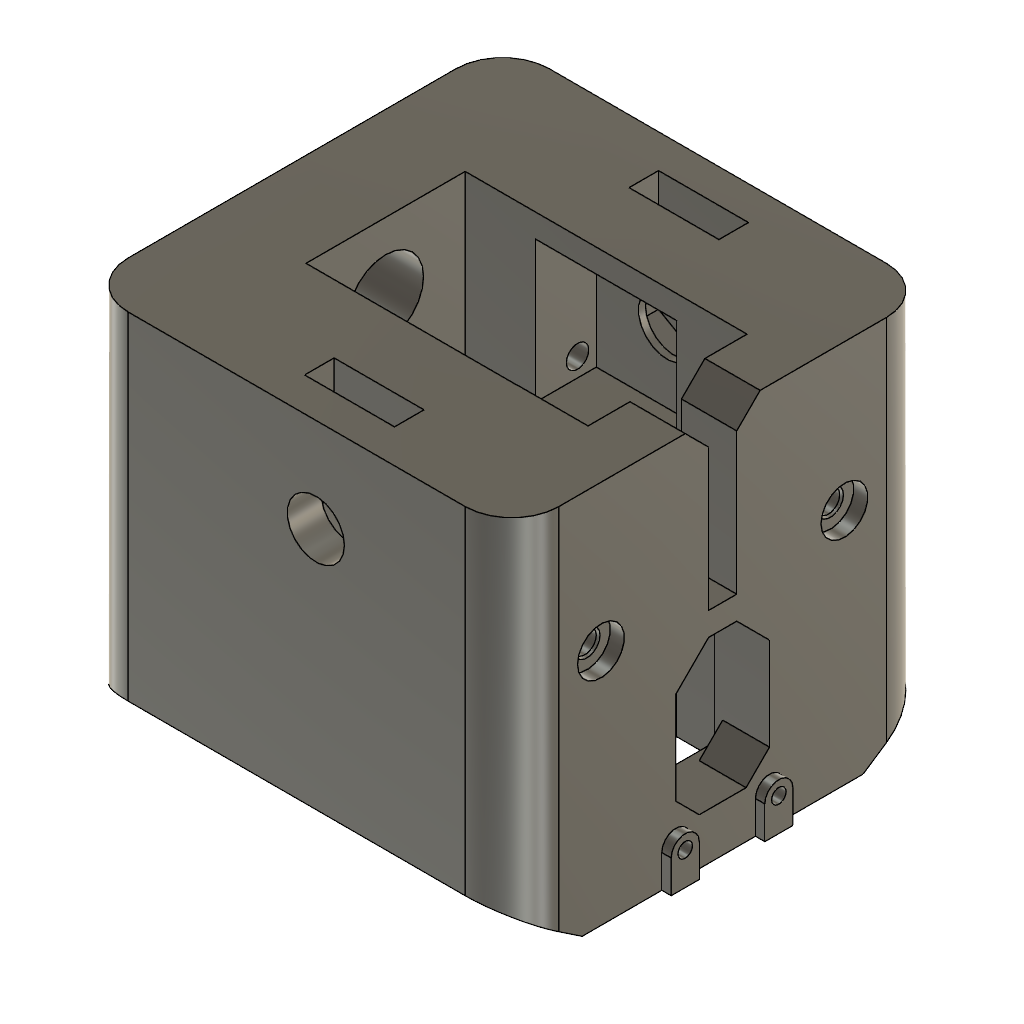
Agarre móvil v40 (Autodesk Fusion 360 design; units mm, degrees)
Autodesk Fusion 360 part; units mm, degrees
sketch "Sketch1" plane through (0, 0, 0) normal (0, 0, 1) x (1, 0, 0)
  line L0 (0, 0) -> (92, 0)
  line L1 (92, 0) -> (92, 60)
  line L2 (92, 60) -> (0, 60)
  line L3 (0, 60) -> (0, 0)
  dimension "d17" = 92
  dimension "d130" = 60
  constraint horizontal L0
  constraint vertical L1
  constraint horizontal L2
  constraint vertical L3
  constraint coincident L0.start L3.end
  measures "d17" distance of L1 L3
  measures "d130" distance of L0 L2
extrude "Extrude1" add sketch "Sketch1" along normal blind 10
sketch "Sketch3" plane through (0, 0, 10) normal (0, 0, 1) x (-1, 0, 0)
  line L0 (0, 0) -> (-92, 0)
  line L1 (-92, 0) -> (-92, -60)
  line L2 (-92, -60) -> (0, -60)
  line L3 (-92, -75) -> (0, -75)
  line L4 (0, -75) -> (0, 15)
  line L5 (0, 15) -> (-92, 15)
  line L6 (-92, 15) -> (-92, -75)
  line L7 (-20, -40) -> (-92, -40)
  line L8 (-92, -40) -> (-92, -20)
  line L9 (-92, -20) -> (-20, -20)
  line L10 (-20, -20) -> (-20, -40)
  line L11 (0, -60) -> (0, 0)
  dimension "d58" = 15
  dimension "d59" = 15
  dimension "d134" = 20
  constraint horizontal L3
  constraint vertical L4
  constraint horizontal L5
  constraint vertical L6
  constraint horizontal L7
  constraint vertical L8
  constraint horizontal L9
  constraint vertical L10
  constraint coincident L6 L8.end
  constraint coincident L1 L8.end
  measures "d58" distance of L2 L3
  measures "d59" distance of L0 L5
  measures "d134" distance of L7 L9
extrude "Extrude3" add sketch "Sketch3" along normal blind 72 contours L0 L1 L2 L4 L6 L7 L9 L10 L11 | L0 L4 L5 L6 | L2 L3 L4 L6
sketch "Sketch4" plane through (20, 0, 0) normal (1, 0, 0) x (0, 1, 0)
  line L0 (20, 82) -> (20, 10)
  line L1 (20, 10) -> (40, 10)
  line L2 (40, 10) -> (40, 82)
  line L3 (40, 82) -> (20, 82)
  circle A0 centre (30, 67) radius 8.1
  dimension "d7" = 16.2
  dimension "d8" = 15
  measures "d7" diameter of A0
  measures "d8" distance of L3 A0.centre
extrude "Extrude4" cut sketch "Sketch4" against normal blind 20 contours A0
sketch "Sketch5" plane through (0, 20, 0) normal (0, 1, 0) x (-1, 0, 0)
  line L0 (-92, 10) -> (-20, 10)
  line L1 (-20, 10) -> (-20, 82)
  line L2 (-20, 82) -> (-92, 82)
  line L3 (-92, 82) -> (-92, 10)
  line L4 (-65.2, 77) -> (-35, 77)
  line L5 (-35, 77) -> (-35, 46.8)
  line L6 (-35, 46.8) -> (-65.2, 46.8)
  line L7 (-65.2, 46.8) -> (-65.2, 77)
  dimension "d11" = 30.2
  dimension "d12" = 30.2
  dimension "d18" = 26.8
  dimension "d67" = 5
  constraint horizontal L4
  constraint vertical L5
  constraint horizontal L6
  constraint vertical L7
  measures "d11" distance of L5 L7
  measures "d12" distance of L4 L6
  measures "d18" distance of L3 L7
  measures "d67" distance of L2 L4
extrude "Extrude5" cut sketch "Sketch5" along normal blind 40 and the other way blind 20 contours L4 L5 L6 L7
sketch "Sketch6" plane through (20, 0, 0) normal (1, 0, 0) x (0, 1, 0)
  circle A0 centre (30, 67) radius 8.1
  line L0 (20, 82) -> (20, 10)
  line L1 (20, 10) -> (40, 10)
  line L2 (40, 10) -> (40, 82)
  line L3 (40, 82) -> (20, 82)
  line L4 (13, 82) -> (47, 82)
  line L5 (47, 82) -> (47, 46.8)
  line L6 (47, 46.8) -> (13, 46.8)
  line L7 (13, 46.8) -> (13, 82)
  dimension "d68" = 35.2
  dimension "d93" = 7
  dimension "d94" = 7
  constraint horizontal L4
  constraint vertical L5
  constraint horizontal L6
  constraint vertical L7
  constraint collinear L3 L4
  measures "d68" distance of L4 L6
  measures "d93" distance of L2 L5
  measures "d94" distance of L0 L7
extrude "Extrude6" cut sketch "Sketch6" along normal blind 45.2 contours L0 L4 L6 L7 | L2 L4 L5 L6
sketch "Sketch7" plane through (65.2, 0, 0) normal (-1, 0, 0) x (0, -1, 0)
  line L0 (-47, 77) -> (-60, 77)
  line L1 (-60, 77) -> (-60, 46.8)
  line L2 (-60, 46.8) -> (-40, 46.8)
  line L3 (-40, 46.8) -> (-40, 82)
  line L4 (-47, 82) -> (-47, 77)
  line L5 (-40, 82) -> (-33, 82)
  line L6 (-33, 82) -> (-33, 46.8)
  line L7 (-33, 46.8) -> (-40, 46.8)
  line L8 (-40, 46.8) -> (-40, 82)
  line L9 (-20, 82) -> (-27, 82)
  line L10 (-27, 82) -> (-27, 46.8)
  line L11 (-27, 46.8) -> (-20, 46.8)
  line L12 (-20, 46.8) -> (-20, 82)
  line L13 (-27, 46.8) -> (-16.8934, 46.8) construction
  line L14 (-20, 10) -> (-20, 82)
  line L15 (-40, 10) -> (-40, 82)
  line L16 (-40, 82) -> (-47, 82)
  line L17 (15, 82) -> (-20, 82)
  line L18 (-20, 46.8) -> (-40, 46.8)
  line L19 (-40, 46.8) -> (-40, 41.8)
  line L20 (-40, 41.8) -> (-20, 41.8)
  line L21 (-20, 41.8) -> (-20, 46.8)
  line L22 (-27, 41.8) -> (-20, 34.8)
  line L23 (-33, 41.8) -> (-40, 34.8)
  dimension "d22" = 7
  dimension "d23" = 7
  dimension "d69" = 35.2
  dimension "d70" = 35.2
  dimension "d101" = 45
  dimension "d102" = 7
  dimension "d103" = 5
  dimension "d104" = 7
  dimension "d131" = 45
  constraint horizontal L5
  constraint vertical L6
  constraint horizontal L7
  constraint vertical L8
  constraint coincident L3.end L5.start
  constraint horizontal L9
  constraint vertical L10
  constraint horizontal L11
  constraint vertical L12
  constraint horizontal L13
  constraint collinear L9 L17
  constraint horizontal L18
  constraint vertical L19
  constraint horizontal L20
  constraint vertical L21
  constraint coincident L15 L19.end
  constraint coincident L14 L22.end
  constraint coincident L20 L22.start
  constraint coincident L20 L23.start
  constraint coincident L15 L23.end
  measures "d22" distance of L10 L12
  measures "d23" distance of L6 L8
  measures "d69" distance of L9.end L10.end
  measures "d70" distance of L5.end L6.end
  measures "d101" angle of L20 L22
  measures "d102" distance of L14 L22.start
  measures "d103" distance of L10.end L20
  measures "d104" distance of L19.end L23.start
  measures "d131" angle of L15 L23
extrude "Extrude7" add sketch "Sketch7" against normal blind 26.8 contours L3 L5 L6 L7 L8 L15 L18 | L7 L11 L14 L15 L18 L19 L20 L21 | L15 L20 L23 | L9 L10 L11 L12 L14 L18 | L14 L20 L22
sketch "Sketch17" plane through (0, 0, 46.8) normal (0, 0, 1) x (-1, 0, 0)
  line L0 (-65.2, -33) -> (-65.2, -27)
  line L1 (-65.2, -27) -> (-92, -27)
  line L2 (-92, -27) -> (-92, -33)
  line L3 (-92, -33) -> (-65.2, -33)
  line L4 (-65.2, -33) -> (-75.2, -33)
  line L5 (-75.2, -33) -> (-75.2, -27)
  line L6 (-75.2, -27) -> (-65.2, -27)
  line L7 (-65.2, -27) -> (-65.2, -33)
  dimension "d105" = 10
  constraint horizontal L4
  constraint vertical L5
  constraint horizontal L6
  constraint vertical L7
  constraint coincident L0.start L3.end
  measures "d105" distance of L0.start L4.end
extrude "Extrude18" cut sketch "Sketch17" against normal blind 6 contours L0 L1 L3 L4 L5 L6 L7
chamfer "Chamfer5" distance 4 angle 45 1 edges at (75.2, 30, 46.8)
sketch "Sketch8" plane through (0, 0, 10) normal (0, 0, 1) x (-1, 0, 0)
  line L0 (-20, -20) -> (-92, -20)
  line L1 (-92, -20) -> (-92, -40)
  line L2 (-92, -40) -> (-20, -40)
  line L3 (-20, -40) -> (-20, -20)
  circle A0 centre (-30, -40) radius 1.6
  circle A1 centre (-50, -40) radius 1.6
  circle A2 centre (-30, -20) radius 1.6
  circle A3 centre (-50, -20) radius 1.6
  dimension "d28" = 3.2
  dimension "d29" = 3.2
  dimension "d30" = 3.2
  dimension "d31" = 3.2
  dimension "d32" = 20
  dimension "d33" = 20
  dimension "d34" = 10
  dimension "d35" = 10
  dimension "d132" = 20
  constraint coincident L2 A0.centre
  constraint coincident L2 A1.centre
  constraint coincident L0 A3.centre
  measures "d28" diameter of A0
  measures "d29" diameter of A1
  measures "d30" diameter of A2
  measures "d31" diameter of A3
  measures "d32" distance of A2.centre A3.centre
  measures "d33" distance of A0.centre A1.centre
  measures "d34" distance of L3 A0.centre
  measures "d35" distance of L3 A2.centre
  measures "d132" distance of A0.centre A2.centre
extrude "Extrude8" cut sketch "Sketch8" against normal blind 10 contours L0 A2 | L0 A2 | L2 A0 | L2 A0 | L0 A3 | L0 A3 | L2 A1 | L2 A1
sketch "Sketch9" plane through (0, 0, 10) normal (0, 0, 1) x (-1, 0, 0)
  arc A0 (-48.4, -40) -> (-51.6, -40) centre (-50, -40) ccw
  line L0 (-48.4, -40) -> (-31.6, -40)
  arc A1 (-28.4, -40) -> (-31.6, -40) centre (-30, -40) ccw
  line L1 (-28.4, -40) -> (-20, -40)
  line L2 (-20, -40) -> (-20, -20)
  line L3 (-20, -20) -> (-28.4, -20)
  arc A2 (-31.6, -20) -> (-28.4, -20) centre (-30, -20) ccw
  line L4 (-31.6, -20) -> (-48.4, -20)
  arc A3 (-51.6, -20) -> (-48.4, -20) centre (-50, -20) ccw
  line L5 (-51.6, -20) -> (-92, -20)
  line L6 (-92, -20) -> (-92, -40)
  line L7 (-92, -40) -> (-51.6, -40)
  circle A4 centre (-30, -40) radius 3
  circle A5 centre (-50, -40) radius 3
  circle A6 centre (-50, -20) radius 3
  circle A7 centre (-30, -20) radius 3
  dimension "d38" = 6
  dimension "d39" = 6
  dimension "d40" = 6
  dimension "d41" = 6
  constraint concentric A1 A4
  constraint concentric A0 A5
  constraint concentric A3 A6
  constraint concentric A2 A7
  measures "d38" diameter of A4
  measures "d39" diameter of A5
  measures "d40" diameter of A6
  measures "d41" diameter of A7
chamfer "Chamfer8" distance 15 distance2 10 2 edges at (46, 0, 10) (46, 60, 10) measured on face at (30.6667, -5, 10) measured on face at (61.3333, 65, 10)
chamfer "Chamfer9" distance 5 angle 45 2 edges at (78.6, 33, 82) (78.6, 27, 82)
extrude "Extrude9" cut sketch "Sketch9" along normal blind 41.8 contours A0 L0 L7 A5 | L0 A1 L1 A4 | L4 A3 L5 A6 | L3 A2 L4 A7 picked at (-50.0747, -40.9972) picked at (-29.9253, -40.9972) picked at (-49.9253, -19.0028) picked at (-29.9253, -19.0028)
sketch "Sketch10" plane through (0, 0, 0) normal (0, 1, 0) x (-1, 0, 0)
  line L0 (-65.2, 46.8) -> (-35, 46.8)
  line L1 (-35, 46.8) -> (-35, 77)
  line L2 (-35, 77) -> (-65.2, 77)
  line L3 (-65.2, 77) -> (-65.2, 46.8)
  circle A0 centre (-50.1, 61.9) radius 6.1
  dimension "d46" = 12.2
  dimension "d47" = 15.1
  dimension "d48" = 15.1
  measures "d46" diameter of A0
  measures "d47" distance of L2 A0.centre
  measures "d48" distance of L3 A0.centre
extrude "Extrude10" cut sketch "Sketch10" along normal blind 75 and the other way blind 15 contours A0
ref_plane "WorkPlane1" through (50.1, -1.5, 61.9) normal (0, 1, 0) x (0, 0, 1)
sketch "Sketch11" plane through (45.1, -1.5, 54.9) normal (0, 1, 0) x (1, 0, 0)
  circle A0 centre (5, -7) radius 6.1
  circle A1 centre (5, -7) radius 6.1
  line L0 (14.6, -1.4574) -> (5, 4.0851)
  line L1 (5, 4.0851) -> (-4.6, -1.4574)
  line L2 (-4.6, -1.4574) -> (-4.6, -12.5426)
  line L3 (-4.6, -12.5426) -> (5, -18.0851)
  line L4 (5, -18.0851) -> (14.6, -12.5426)
  line L5 (14.6, -12.5426) -> (14.6, -1.4574)
  line L6 (14.6, -1.4574) -> (-4.6, -1.4574)
  line L7 (-4.6, -1.4574) -> (-4.6, -28.6763)
  line L8 (-4.6, -28.6763) -> (14.6, -28.6763)
  line L9 (14.6, -28.6763) -> (14.6, -1.4574)
  point P0 (5, -7)
  point P1 (5, -7)
  point P2 (5, -7)
  point P3 (5, -7)
  dimension "d128" = 9.6
  constraint coincident P3 P0
  constraint coincident P1 P0
  constraint coincident P2 P1
  constraint horizontal L6
  constraint vertical L7
  constraint horizontal L8
  constraint vertical L9
  measures "d128" distance of P3 L5
extrude "Extrude11" cut sketch "Sketch11" against normal blind 6.3
ref_plane "WorkPlane2" through (50.1, 61.5, 61.9) normal (0, -1, 0) x (0, 0, -1)
sketch "Sketch12" plane through (45.1, 61.5, 54.9) normal (0, -1, 0) x (1, 0, 0)
  circle A0 centre (5, 7) radius 6.1
  line L0 (14.6, 12.5426) -> (5, 18.0851)
  line L1 (5, 18.0851) -> (-4.6, 12.5426)
  line L2 (-4.6, 12.5426) -> (-4.6, 1.4574)
  line L3 (-4.6, 1.4574) -> (5, -4.0851)
  line L4 (5, -4.0851) -> (14.6, 1.4574)
  line L5 (14.6, 1.4574) -> (14.6, 12.5426)
  line L6 (-4.6, 1.4574) -> (14.6, 1.4574)
  line L7 (14.6, 1.4574) -> (14.6, 28.1341)
  line L8 (14.6, 28.1341) -> (-4.6, 28.1341)
  line L9 (-4.6, 28.1341) -> (-4.6, 1.4574)
  point P0 (5, 7)
  point P1 (5, 7)
  dimension "d95" = 9.6
  constraint coincident P0 A0.centre
  constraint coincident P1 P0
  constraint horizontal L6
  constraint vertical L7
  constraint horizontal L8
  constraint vertical L9
  measures "d95" distance of P1 L5
extrude "Extrude12" cut sketch "Sketch12" against normal blind 6.3 contours A0 L0 L1 L2 L5 L6 L7 L9 | A0 L3 L4 L6 | L0 L1 L7 L8 L9
sketch "Sketch13" plane through (92, 0, 0) normal (1, 0, 0) x (0, 1, 0)
  line L0 (75, 82) -> (38, 82)
  line L1 (40, 34.8) -> (40, 10)
  line L2 (40, 10) -> (20, 10)
  line L3 (20, 10) -> (20, 34.8)
  line L4 (0, 0) -> (60, 0)
  circle A0 centre (20, 7) radius 1.55
  circle A1 centre (40, 7) radius 1.55
  circle A2 centre (20, 7) radius 3
  circle A3 centre (40, 7) radius 3
  line L5 (17, 7) -> (17, 0)
  line L6 (23, 7) -> (23, 0)
  line L7 (37, 7) -> (37, 0)
  line L8 (43, 7) -> (43, 0)
  line L9 (33, 77) -> (33, 46.8)
  line L10 (27, 46.8) -> (27, 77)
  line L11 (33, 46.8) -> (27, 46.8)
  line L12 (20, 34.8) -> (27, 41.8)
  line L13 (27, 41.8) -> (33, 41.8)
  line L14 (33, 41.8) -> (40, 34.8)
  line L15 (22, 82) -> (-15, 82)
  line L16 (-15, 82) -> (-15, 10)
  line L17 (75, 10) -> (75, 82)
  line L18 (27, 77) -> (22, 82)
  line L19 (-15, 10) -> (0, 0)
  line L20 (60, 0) -> (75, 10)
  line L21 (38, 82) -> (33, 77)
  dimension "d71" = 3.1
  dimension "d72" = 3.1
  dimension "d73" = 20
  dimension "d74" = 7
  dimension "d75" = 6
  dimension "d76" = 6
  constraint concentric A0 A2
  constraint concentric A1 A3
  constraint coincident A2 L5.start
  constraint coincident L4 L5.end
  constraint tangent A2 L5
  constraint perpendicular L4 L5
  constraint coincident A2 L6.start
  constraint coincident L4 L6.end
  constraint tangent A2 L6
  constraint perpendicular L4 L6
  constraint coincident L4 L7.end
  constraint perpendicular L4 L7
  constraint coincident A3 L8.start
  constraint coincident L4 L8.end
  constraint tangent A3 L8
  constraint perpendicular L4 L8
  constraint coincident A3 L7.start
  measures "d71" diameter of A0
  measures "d72" diameter of A1
  measures "d73" distance of A0.centre A1.centre
  measures "d74" distance of L4 A0.centre
  measures "d75" diameter of A2
  measures "d76" diameter of A3
extrude "Extrude13" add sketch "Sketch13" along normal blind 2 contours L4 A3 L7 L8 | A3 | L4 A2 L5 L6 | A2
extrude "Extrude14" cut 2 faces at (92, 20.1888, 7.481) (92, 39.3809, 6.5283) along direction (-1, 0, 0) blind 7
sketch "Sketch15" plane through (92, 0, 0) normal (1, 0, 0) x (0, 1, 0)
  line L0 (17, 0) -> (17, 7)
  arc A0 (20, 10) -> (17, 7) centre (20, 7) ccw
  line L1 (20, 10) -> (20, 34.8)
  line L2 (75, 82) -> (38, 82)
  line L3 (43, 0) -> (60, 0)
  line L4 (37, 0) -> (37, 7)
  arc A1 (40, 10) -> (37, 7) centre (40, 7) ccw
  line L5 (40, 10) -> (20, 10)
  arc A2 (23, 7) -> (20, 10) centre (20, 7) ccw
  line L6 (23, 7) -> (23, 0)
  line L7 (23, 0) -> (37, 0)
  line L8 (43, 7) -> (43, 0)
  line L9 (43, 0) -> (60, 0)
  line L10 (75, 82) -> (38, 82)
  line L11 (40, 34.8) -> (40, 10)
  arc A3 (43, 7) -> (40, 10) centre (40, 7) ccw
  line L12 (20, 15) -> (25, 10)
  line L13 (20, 15) -> (27.0711, 15) construction
  line L14 (40, 15) -> (35, 10)
  line L15 (27, 46.8) -> (27, 77)
  line L16 (33, 77) -> (33, 46.8)
  line L17 (43, 7) -> (43, 0)
  line L18 (33, 77) -> (33, 46.8)
  line L19 (33, 46.8) -> (27, 46.8)
  line L20 (40, 34.8) -> (40, 10)
  arc A4 (43, 7) -> (40, 10) centre (40, 7) ccw
  line L21 (33, 46.8) -> (27, 46.8)
  line L22 (27, 46.8) -> (27, 77)
  line L23 (17, 0) -> (17, 7)
  arc A5 (20, 10) -> (17, 7) centre (20, 7) ccw
  line L24 (20, 10) -> (20, 34.8)
  line L25 (20, 34.8) -> (27, 41.8)
  line L26 (20, 34.8) -> (27, 41.8)
  line L27 (27, 41.8) -> (33, 41.8)
  line L28 (33, 41.8) -> (40, 34.8)
  line L29 (27, 41.8) -> (33, 41.8)
  line L30 (33, 41.8) -> (40, 34.8)
  line L31 (75, 10) -> (75, 82)
  line L32 (22, 82) -> (-15, 82)
  line L33 (-15, 82) -> (-15, 10)
  line L34 (75, 10) -> (75, 82)
  line L35 (22, 82) -> (-15, 82)
  line L36 (-15, 82) -> (-15, 10)
  line L37 (60, 0) -> (75, 10)
  line L38 (38, 82) -> (33, 77)
  line L39 (27, 77) -> (22, 82)
  line L40 (-15, 10) -> (0, 0)
  line L41 (0, 0) -> (17, 0)
  line L42 (60, 0) -> (75, 10)
  line L43 (38, 82) -> (33, 77)
  line L44 (27, 77) -> (22, 82)
  line L45 (-15, 10) -> (0, 0)
  line L46 (0, 0) -> (17, 0)
  dimension "d86" = 45
  constraint horizontal L13
  constraint coincident L1 L12.start
  constraint coincident L5 L12.end
  constraint coincident L11 L14.start
  constraint coincident L5 L14.end
  constraint perpendicular L12 L14
  measures "d86" angle of L12 L13
extrude "Extrude16" add sketch "Sketch15" against normal blind 10 contours L1 L5 L12 L24 | L5 L11 L14 L20
ref_plane "WorkPlane3" through (86, 20, 7) normal (1, 0, 0) x (0, 1, 0)
sketch "Sketch14" plane through (86, 20, 7) normal (1, 0, 0) x (0, 1, 0)
  line L0 (2.85, 1.6454) -> (0, 3.2909)
  line L1 (0, 3.2909) -> (-2.85, 1.6454)
  line L2 (-2.85, 1.6454) -> (-2.85, -1.6454)
  line L3 (-2.85, -1.6454) -> (0, -3.2909)
  line L4 (0, -3.2909) -> (2.85, -1.6454)
  line L5 (2.85, -1.6454) -> (2.85, 1.6454)
  line L6 (17.1705, -1.6805) -> (20.0406, -3.2906)
  line L7 (20.0406, -3.2906) -> (22.8701, -1.6102)
  line L8 (22.8701, -1.6102) -> (22.8295, 1.6805)
  line L9 (22.8295, 1.6805) -> (19.9594, 3.2906)
  line L10 (19.9594, 3.2906) -> (17.1299, 1.6102)
  line L11 (17.1299, 1.6102) -> (17.1705, -1.6805)
  line L12 (-2.85, -1.6454) -> (-2.85, -7)
  line L13 (2.85, -1.6454) -> (2.85, -7)
  line L14 (17.1705, -1.6805) -> (22.8498, -1.6805)
  line L15 (22.8498, -1.6805) -> (22.8498, -7.3381)
  line L16 (22.8498, -7.3381) -> (17.1705, -7.3381)
  line L17 (17.1705, -7.3381) -> (17.1705, -1.6805)
  line L18 (2.85, -7) -> (-2.85, -7)
  point P0 (20, 0)
  dimension "d82" = 2.85
  dimension "d83" = 2.85
  constraint parallel L2 L12
  constraint parallel L5 L13
  constraint horizontal L14
  constraint vertical L15
  constraint horizontal L16
  constraint vertical L17
  constraint perpendicular L12 L18
  measures "d82" distance of origin L5
  measures "d83" distance of P0 L11
extrude "Extrude15" cut sketch "Sketch14" along normal blind 2.6
sketch "Sketch16" plane through (20, 0, 0) normal (1, 0, 0) x (0, 1, 0)
  circle A0 centre (30, 67) radius 8.1
  line L0 (20, 46.8) -> (20, 10)
  line L1 (20, 10) -> (40, 10)
  line L2 (40, 10) -> (40, 46.8)
  line L3 (40, 46.8) -> (47, 46.8)
  line L4 (47, 46.8) -> (47, 82)
  line L5 (47, 82) -> (13, 82)
  line L6 (13, 82) -> (13, 46.8)
  circle A1 centre (30, 30) radius 7
  line L7 (60, 0) -> (0, 0)
  line L8 (13, 46.8) -> (20, 46.8)
  dimension "d89" = 14
  dimension "d90" = 30
  measures "d89" diameter of A1
  measures "d90" distance of A1.centre L7
extrude "Extrude17" cut sketch "Sketch16" against normal blind 20 contours A1
chamfer "Chamfer3" distance 7 angle 45 2 edges at (65.2, 40, 40.8) (65.2, 20, 40.8)
sketch "Sketch18" plane through (0, 0, 0) normal (-1, 0, 0) x (0, -1, 0)
  circle A0 centre (-30, 30) radius 7
  circle A1 centre (-30, 67) radius 8.1
  line L0 (15, 82) -> (-75, 82)
  line L1 (-60, 0) -> (0, 0)
  circle A2 centre (-56, 50.8) radius 2.4
  circle A3 centre (-4, 50.8) radius 2.4
  line L2 (-20, 46.8) -> (-17, 46.8)
  line L3 (-20, 46.8) -> (-13, 46.8)
  line L4 (-13, 46.8) -> (0, 46.8)
  line L5 (0, 46.8) -> (-27, 46.8)
  line L6 (-27, 46.8) -> (-20, 46.8)
  line L7 (-20, 46.8) -> (-17, 46.8)
  line L8 (-43, 46.8) -> (-40, 46.8)
  line L9 (-40, 46.8) -> (-33, 46.8)
  line L10 (-33, 46.8) -> (-60, 46.8)
  line L11 (-60, 46.8) -> (-47, 46.8)
  line L12 (-47, 46.8) -> (-40, 46.8)
  line L13 (-43, 46.8) -> (-40, 46.8)
  line L14 (15, 10) -> (15, 82)
  line L15 (-75, 82) -> (-75, 10)
  line L16 (0, 0) -> (15, 10)
  line L17 (-75, 10) -> (-60, 0)
  dimension "d109" = 4.8
  dimension "d110" = 4.8
  dimension "d123" = 4
  dimension "d124" = 4
  dimension "d140" = 19
  dimension "d141" = 19
  measures "d109" diameter of A2
  measures "d110" diameter of A3
  measures "d123" distance of A2.centre L11
  measures "d124" distance of A3.centre L5
  measures "d140" distance of A3.centre L14
  measures "d141" distance of A2.centre L15
extrude "Extrude19" cut sketch "Sketch18" against normal blind 92 contours A2 | A3
sketch "Sketch20" plane through (92, 0, 0) normal (1, 0, 0) x (0, 1, 0)
  circle A0 centre (4, 50.8) radius 2.4
  circle A1 centre (56, 50.8) radius 2.4
  arc A2 (43, 7) -> (37, 7) centre (40, 7) ccw
  line L0 (43, 7) -> (43, 0)
  line L1 (43, 0) -> (60, 0)
  line L2 (75, 82) -> (38, 82)
  line L3 (33, 77) -> (33, 46.8)
  line L4 (33, 46.8) -> (27, 46.8)
  line L5 (27, 46.8) -> (27, 77)
  line L6 (17, 0) -> (17, 7)
  arc A3 (23, 7) -> (17, 7) centre (20, 7) ccw
  line L7 (23, 7) -> (23, 0)
  line L8 (23, 0) -> (37, 0)
  line L9 (37, 0) -> (37, 7)
  line L10 (40, 15) -> (35, 10)
  line L11 (35, 10) -> (25, 10)
  line L12 (25, 10) -> (20, 15)
  line L13 (20, 15) -> (20, 34.8)
  line L14 (20, 34.8) -> (27, 41.8)
  line L15 (27, 41.8) -> (33, 41.8)
  line L16 (33, 41.8) -> (40, 34.8)
  line L17 (40, 34.8) -> (40, 15)
  circle A4 centre (4, 50.8) radius 5
  circle A5 centre (56, 50.8) radius 5
  line L18 (75, 10) -> (75, 82)
  line L19 (22, 82) -> (-15, 82)
  line L20 (-15, 82) -> (-15, 10)
  line L21 (60, 0) -> (75, 10)
  line L22 (38, 82) -> (33, 77)
  line L23 (27, 77) -> (22, 82)
  line L24 (-15, 10) -> (0, 0)
  line L25 (0, 0) -> (17, 0)
  dimension "d125" = 10
  dimension "d126" = 10
  constraint concentric A0 A4
  constraint concentric A1 A5
  measures "d125" diameter of A4
  measures "d126" diameter of A5
extrude "Extrude20" cut sketch "Sketch20" against normal blind 3 contours A4 | A5
chamfer "Chamfer6" distance 0.4 angle 45 2 edges at (89, 6.2376, 51.6679) (89, 58.2376, 51.6679)
chamfer "Chamfer7" distance 0.6 angle 45 8 edges at (86, 20, 0) (87.3, 22.85, 0) (88.6, 20, 0) (87.3, 17.15, 0) (88.6, 40.0101, 0) (86, 40.0101, 0) (87.3, 37.1705, 0) (87.3, 42.8498, 0)
fillet "Fillet2" radius 10 4 edges at (92, -15, 46) (92, 75, 46) (0, 75, 46) (0, -15, 46)
sketch "Boceto21" plane through (0, 0, 82) normal (0, 0, 1) x (-1, 0, 0)
  arc A0 (0, 5) -> (-10, 15) centre (-10, 5) ccw
  line L0 (-10, 15) -> (-82, 15)
  arc A1 (-82, 15) -> (-92, 5) centre (-82, 5) ccw
  line L1 (-92, 5) -> (-92, -22)
  line L2 (-92, -22) -> (-65.2, -22)
  line L3 (-65.2, -22) -> (-65.2, -13)
  line L4 (-65.2, -13) -> (-20, -13)
  line L5 (-20, -13) -> (-20, -47)
  line L6 (-20, -47) -> (-65.2, -47)
  line L7 (-65.2, -47) -> (-65.2, -38)
  line L8 (-65.2, -38) -> (-92, -38)
  line L9 (-92, -38) -> (-92, -65)
  arc A2 (-92, -65) -> (-82, -75) centre (-82, -65) ccw
  line L10 (-82, -75) -> (-10, -75)
  arc A3 (-10, -75) -> (0, -65) centre (-10, -65) ccw
  line L11 (0, -65) -> (0, 5)
  line L12 (-40.5, -61.5) -> (-40.5, -67.8)
  line L13 (-40.5, -67.8) -> (-59.7, -67.8)
  line L14 (-59.7, -67.8) -> (-59.7, -61.5)
  line L15 (-59.7, -61.5) -> (-40.5, -61.5)
  line L16 (-59.7, 1.5) -> (-59.7, 7.8)
  line L17 (-59.7, 7.8) -> (-40.5, 7.8)
  line L18 (-40.5, 7.8) -> (-40.5, 1.5)
  line L19 (-40.5, 1.5) -> (-59.7, 1.5)
  line L20 (-65.2, -47) -> (-80.2, -47)
  line L21 (-80.2, -47) -> (-80.2, -13.0418)
  line L22 (-80.2, -13.0418) -> (-65.2, -13.0418)
  line L23 (-65.2, -13.0418) -> (-65.2, -47)
  dimension "d142" = 15
  constraint horizontal L20
  constraint vertical L21
  constraint horizontal L22
  constraint vertical L23
  constraint coincident L6.end L7.start
  measures "d142" distance of L6.end L20.end
extrude "Extruir21" cut sketch "Boceto21" along normal through all and the other way through all contours L2 L3 L21 L22 L23 | L2 L8 L21 L23 | L7 L8 L20 L21 L23
